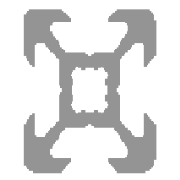
# Autodesk Inventor part: 2020 V-slot 100mm
Saved by Autodesk Inventor 2023 (Build 270158000, 158)
## iProperties
Created: 2023-08-13
Part Number: 2020 V-slot 100mm
Material: Generic
Description: STEP AP214
Document SubType Name: Modeling
Designer: Felix
Language: en-US
Size Designation: (Unnamed 1)
Categories: <MemberInstance><Categories><Category DisplayName="Structural Shapes" InternalName="089c4875-fa83-4c05-b084-43b9cc11f5ed" Mnemonic="GRDR"><CategoryParameter DisplayName="Mass per Length Unit" InternalName="0bb95a10-148f-4027-a459-38d7b056702a" Mnemonic="shpmass"/><CategoryParameter DisplayName="Section Area" InternalName="1ff91680-64b0-4202-b9a3-7fd3f94bba3b" Mnemonic="secarea"/><CategoryParameter DisplayName="Radius of Gyration (x)" InternalName="25778675-03e9-40c1-b6a8-4a9ed693320d" Mnemonic="gyrradx"/><CategoryParameter DisplayName="Torsional Rigidity Modulus" InternalName="26c1ec35-5026-4c63-ad0a-751cf684a536" Mnemonic="torrigmod"/><CategoryParameter DisplayName="Distance of the Center of Gravity X-X" InternalName="26c9bdb8-9c79-4b4f-a92e-8e197583c9c4" Mnemonic="grcendistX"/><CategoryParameter DisplayName="Legacy Member ID" InternalName="340afe4f-75d7-48d3-ab7d-943f3c3da468" Mnemonic="LegacyMemberID"/><CategoryParameter DisplayName="Base Length" InternalName="42e34263-8f20-4d0e-ad48-bf1385b87c24" Mnemonic="shplen"/><CategoryParameter DisplayName="Moment of Inertia (y)" InternalName="4b9f58ea-bced-460e-81ea-3d29ca5a49e3" Mnemonic="inermomy"/><CategoryParameter DisplayName="Moment of Inertia (x)" InternalName="4cd780bc-73d7-43ac-917a-579e5cbd684d" Mnemonic="inermomx"/><CategoryParameter DisplayName="Custom Base Point" InternalName="4f1d1b73-316d-484b-a3df-9cbabb16eb77" Mnemonic="shpBasePoint"/><CategoryParameter DisplayName="Shape Height" InternalName="50274e7d-5ac0-4796-92cb-c59e54983c67" Mnemonic="shpheig"/><CategoryParameter DisplayName="Section Module (y)" InternalName="59eaa5e9-d227-48dc-b6c1-6920f96e0f95" Mnemonic="secmody"/><CategoryParameter DisplayName="Section Designation" InternalName="5a64d034-428d-49c8-ba32-7619764de20f" Mnemonic="shpdes"/><CategoryParameter DisplayName="Section Module (x)" InternalName="72cfad18-cf51-4ed4-aaa7-c6b224f8419f" Mnemonic="secmodx"/><CategoryParameter DisplayName="Torsional Section Modulus" InternalName="7c55a8dc-8844-49f9-a867-cc677b30ec9a" Mnemonic="torsecmod"/><CategoryParameter DisplayName="Shape Width" InternalName="7c717d54-a18f-4666-b4d4-573cce22c62c" Mnemonic="shpwdth"/><CategoryParameter DisplayName="Second Shape Thickness" InternalName="9251a8e1-85fd-4e47-af99-afdb762317d9" Mnemonic="shpthick2"/><CategoryParameter DisplayName="FG Authored" InternalName="9c666724-f362-4ea7-ac62-f6a007de5c69" Mnemonic="shpFGAuto"/><CategoryParameter DisplayName="Distance of the Center of Gravity Y-Y" InternalName="bcc4fb17-7af4-436a-8f8c-d0aa3b0248c5" Mnemonic="grcendistY"/><CategoryParameter DisplayName="Radius of Gyration (y)" InternalName="bfa18ebe-1636-4dbe-8d42-b263e0b73184" Mnemonic="gyrrady"/><CategoryParameter DisplayName="Shape Thickness" InternalName="d109cf76-8eb4-42fc-9800-4409734adc67" Mnemonic="shpthick"/><CategoryParameter DisplayName="Coefficient of Shear Displacement" InternalName="de4c90c6-aaa8-468f-a335-6737b311b5d3" Mnemonic="shdispc"/><Category DisplayName="Other" InternalName="f02205ff-2390-476f-921c-0b3185f88e84" Mnemonic="OTHSHP"><CategoryParameter DisplayName="Moment of Inertia (y)" InternalName="044c654e-f649-48ac-84cc-650a29ae31ca" Mnemonic="inermomy"/><CategoryParameter DisplayName="Shape Thickness" InternalName="12b1a788-9233-48fd-a933-2df8ff42b15f" Mnemonic="shpthick"/><CategoryParameter DisplayName="Mass per Length Unit" InternalName="2fd289d6-9394-4d2d-97e6-6659d7d4551d" Mnemonic="shpmass"/><CategoryParameter DisplayName="Radius of Gyration (y)" InternalName="743e1dfe-1bba-408b-b985-cf752b207386" Mnemonic="gyrrady"/><CategoryParameter DisplayName="Section Module (y)" InternalName="88b8bff9-a616-4028-93d5-ed4f79680d13" Mnemonic="secmody"/><CategoryParameter DisplayName="Section Area" InternalName="c46ecdf8-b6eb-4db9-8b25-30258930c1e3" Mnemonic="secarea"/><CategoryParameter DisplayName="Section Module (x)" InternalName="cac70804-9d39-43bb-be17-56ea1f39a6c2" Mnemonic="secmodx"/><CategoryParameter DisplayName="Moment of Inertia (x)" InternalName="ec6737bc-264f-43ed-b0bd-f6d410c2718d" Mnemonic="inermomx"/><CategoryParameter DisplayName="Radius of Gyration (x)" InternalName="ee72c61e-565e-4fd6-b448-66e1e1abcb7e" Mnemonic="gyrradx"/></Category></Category><Category DisplayName="DataType" InternalName="23b78d0f-2648-40c6-8793-ca6db495c9e8" Mnemonic="DATATYPE"><CategoryParameter DisplayName="DisplayName" InternalName="05415f3d-3907-474b-a020-eb9d644f4cf3" Mnemonic="DISPLAYNAME"/><CategoryParameter DisplayName="Standard" InternalName="0c0a119c-1e12-4c84-803f-101930972f5e" Mnemonic="STANDARD"/><CategoryParameter DisplayName="Description" InternalName="13903e3d-64b1-4950-80da-f627842ea37f" Mnemonic="DESCRIPTION"/><CategoryParameter DisplayName="Designation" InternalName="2675968c-4ce5-49e0-a4f5-552d29089031" Mnemonic="DESIGNATION"/><CategoryParameter DisplayName="Default Row" InternalName="2af9ec52-faaa-4026-b378-f9fa4afca842" Mnemonic="DEFAULTROW"/><CategoryParameter DisplayName="Folder Name" InternalName="3f06958e-8713-4116-9be7-ed6184ecc97b" Mnemonic="FOLDERNAME"/><CategoryParameter DisplayName="Revision Guid" InternalName="45a75005-10b1-4dfc-8d6d-dfe629f0b93c" Mnemonic="REVISIONGUID"/><CategoryParameter DisplayName="FileName" InternalName="8b46a4cc-9585-4fed-90c3-899f57e09a73" Mnemonic="FILENAME"/><CategoryParameter DisplayName="StdsOrg" InternalName="8f5914e1-4693-403f-8ab5-d37768198c9d" Mnemonic="STDSORG"/><CategoryParameter DisplayName="Family Version" InternalName="914462f6-6e19-4b14-ba84-155b9680b1d0" Mnemonic="FAMILYREVISION"/><CategoryParameter DisplayName="Standard Revision" InternalName="91d5a463-65c2-4fde-b823-3b7fea5e8e17" Mnemonic="STANDARDREVISION"/><CategoryParameter DisplayName="Member Revision" InternalName="a65d44b9-392f-4f4f-857b-e4b3d54996fe" Mnemonic="MEMBERREVISION"/><CategoryParameter DisplayName="ClipFormat" InternalName="bc51e27b-3422-4e78-93ef-cec197ddf230" Mnemonic="CLIPFORMAT"/><CategoryParameter DisplayName="Manufacturer" InternalName="cd6c7a72-a28a-4e50-99a9-2c7f4e13e5ad" Mnemonic="MANUFACTURER"/><CategoryParameter DisplayName="InternalName" InternalName="cf1d0246-76d9-4b4a-8305-fa0409afb5c1" Mnemonic="INTERNALNAME"/><CategoryParameter DisplayName="IsMetric" InternalName="e2385c5b-1ea4-4823-96a8-8de651266ec3" Mnemonic="ISMETRIC"/><Category DisplayName="Part" InternalName="c0e0b642-3bcb-4cc8-9e80-f96d35c4afa4" Mnemonic="PART"><CategoryParameter DisplayName="Part Number" InternalName="016b6077-bfbe-49bd-92c9-d8d59c39c941" Mnemonic="PARTNUMBER"/><CategoryParameter DisplayName="Stock Number" InternalName="4dba7c1c-e26c-444e-836c-b08b433409a8" Mnemonic="STOCKNUMBER"/><CategoryParameter DisplayName="Material Key" InternalName="5c9a8adb-dd2b-4535-b97f-0a94a95fe41f" Mnemonic="MATERIALKEY"/><CategoryParameter DisplayName="Material" InternalName="818a152a-d3c3-49ca-80ee-df7d91421b8e" Mnemonic="MATERIAL"/></Category></Category></Categories><FamilyTemplate Id="3663_20220714183005_2020 V-slot 100mm"><FamilyTemplateParameters><FamilyTemplateParameter ObjectType="kUserParameterObject" ValueType="xs:double" Id="12" ObjectReferenceKey="LENGTH"/><FamilyTemplateParameter ObjectType="kPartComponentDefinitionObject" ValueType="xs:string" Id="23" SubObjectId="Material"/><FamilyTemplateParameter ObjectType="kPropertyObject" ValueType="xs:string" Id="26" ObjectReferenceKey="{32853F0F-3444-11d1-9E93-0060B03C1CA6}" SubObjectId="5"/><FamilyTemplateParameter ObjectType="kPropertyObject" ValueType="xs:string" Id="27" ObjectReferenceKey="{32853F0F-3444-11d1-9E93-0060B03C1CA6}" SubObjectId="52"/></FamilyTemplateParameters></FamilyTemplate><CategoryParameterMap><ParamToTemplateMap><ParamToTemplate CategoryParameter="//CategoryParameter[@InternalName='cf1d0246-76d9-4b4a-8305-fa0409afb5c1']" ConstantValue="2063e620-472c-4390-8693-845126e34f3a"/><ParamToTemplate CategoryParameter="//CategoryParameter[@InternalName='45a75005-10b1-4dfc-8d6d-dfe629f0b93c']" ConstantValue="7112f66b-08bf-44d2-881c-74bfb6beee39"/><ParamToTemplate CategoryParameter="//CategoryParameter[@InternalName='3f06958e-8713-4116-9be7-ed6184ecc97b']" ConstantValue="2020 V-slot"/><ParamToTemplate CategoryParameter="//CategoryParameter[@InternalName='8f5914e1-4693-403f-8ab5-d37768198c9d']" TemplateParameter="17"/><ParamToTemplate CategoryParameter="//CategoryParameter[@InternalName='0c0a119c-1e12-4c84-803f-101930972f5e']" TemplateParameter="18"/><ParamToTemplate CategoryParameter="//CategoryParameter[@InternalName='91d5a463-65c2-4fde-b823-3b7fea5e8e17']" TemplateParameter="19"/><ParamToTemplate CategoryParameter="//CategoryParameter[@InternalName='cd6c7a72-a28a-4e50-99a9-2c7f4e13e5ad']" TemplateParameter="20"/><ParamToTemplate CategoryParameter="//CategoryParameter[@InternalName='13903e3d-64b1-4950-80da-f627842ea37f']" ConstantValue="STEP AP214"/><ParamToTemplate CategoryParameter="//CategoryParameter[@InternalName='05415f3d-3907-474b-a020-eb9d644f4cf3']" ConstantValue="2020 V-slot"/><ParamToTemplate CategoryParameter="//CategoryParameter[@InternalName='914462f6-6e19-4b14-ba84-155b9680b1d0']" ConstantValue="11"/><ParamToTemplate CategoryParameter="//CategoryParameter[@InternalName='bc51e27b-3422-4e78-93ef-cec197ddf230']" ConstantValue="CF_INVENTOR.STDPARTS"/><ParamToTemplate CategoryParameter="//CategoryParameter[@InternalName='e2385c5b-1ea4-4823-96a8-8de651266ec3']" ConstantValue="true"/><ParamToTemplate CategoryParameter="//CategoryParameter[@InternalName='2af9ec52-faaa-4026-b378-f9fa4afca842']" ConstantValue="1"/><ParamToTemplate CategoryParameter="//CategoryParameter[@InternalName='9c666724-f362-4ea7-ac62-f6a007de5c69']" ConstantValue="1"/><ParamToTemplate CategoryParameter="//CategoryParameter[@InternalName='8b46a4cc-9585-4fed-90c3-899f57e09a73']" ConstantValue="1"/><ParamToTemplate CategoryParameter="//CategoryParameter[@InternalName='a65d44b9-392f-4f4f-857b-e4b3d54996fe']" ConstantValue="1e38da75-13bc-491b-9e5a-c7c1421ad0a4"/><ParamToTemplate CategoryParameter="//CategoryParameter[@InternalName='a65d44b9-392f-4f4f-857b-e4b3d54996fe']" ConstantValue="1e38da75-13bc-491b-9e5a-c7c1421ad0a4"/><ParamToTemplate CategoryParameter="//CategoryParameter[@InternalName='2675968c-4ce5-49e0-a4f5-552d29089031']" TemplateParameter="27"/><ParamToTemplate CategoryParameter="//CategoryParameter[@InternalName='42e34263-8f20-4d0e-ad48-bf1385b87c24']" TemplateParameter="12"/><ParamToTemplate CategoryParameter="//CategoryParameter[@InternalName='818a152a-d3c3-49ca-80ee-df7d91421b8e']" TemplateParameter="23"/><ParamToTemplate CategoryParameter="//CategoryParameter[@InternalName='016b6077-bfbe-49bd-92c9-d8d59c39c941']" TemplateParameter="26"/></ParamToTemplateMap></CategoryParameterMap></MemberInstance>
Density: 1 g/cm^3
Appearance: Default
IsCustomPart: 1
_CCFamilyDisplayName: 2020 V-slot - STEP AP214
_FrameMemberDoc: Frame Member File
_Version: 25.0.0
_GetPNFromCC: 1
Title: 2020 V-slot 100mm.STEP
Author: Felix
Sending System: SolidWorks 2018
Preprocessor: SwSTEP 2.0
G_L: 520,000 mm
G_W: 20,000 mm
G_H: 20,000 mm
+3BCE196E-394D-4133-8DB2-D45BFDC7B2EE+CUTDETAIL1: Corner Joint
+C0951EA9-A871-42D9-A546-154018CCC8EC+CUTDETAIL2: Corner Joint
Autodesk Inventor part; units mm, degrees
ref_plane "YZ Plane" through (0, 0, 0) normal (1, 0, 0) x (0, 1, 0)
ref_plane "XZ Plane" through (0, 0, 0) normal (0, 1, 0) x (-1, 0, 0)
ref_plane "XY Plane" through (0, 0, 0) normal (0, 0, 1) x (1, 0, 0)
ref_plane "Work Plane5" through (12.8, 0, 50) normal (0, 0, 1) x (1, 0, 0)
sketch "Sketch" plane through (12.8, 0, 50) normal (0, 0, 1) x (1, 0, 0)
  arc A0 (1.7, 2.7322) -> (1.5536, 3.0858) centre (1.2, 2.7322) ccw
  line L0 (1.7, 2.7322) -> (1.7, 2)
  arc A1 (1.2, 1.5) -> (1.7, 2) centre (1.2, 2) ccw
  line L1 (1.2, 1.5) -> (-1.2, 1.5)
  line L2 (-1.2, 1.5) -> (-1.2, 1.2)
  line L3 (-1.2, 1.2) -> (0, 0)
  line L4 (0, 0) -> (4.2, 0)
  arc A2 (4.2, 0) -> (5.7, 1.5) centre (4.2, 1.5) ccw
  line L5 (5.7, 1.5) -> (5.7, 5.7)
  line L6 (5.7, 5.7) -> (4.5, 6.9)
  line L7 (4.5, 6.9) -> (4.2, 6.9)
  line L8 (4.2, 6.9) -> (4.2, 4.5)
  arc A3 (3.7, 4) -> (4.2, 4.5) centre (3.7, 4.5) ccw
  line L9 (3.7, 4) -> (2.9678, 4)
  arc A4 (2.6142, 4.1464) -> (2.9678, 4) centre (2.9678, 4.5) ccw
  line L10 (2.6142, 4.1464) -> (0.3464, 6.4142)
  arc A5 (0.2, 6.7678) -> (0.3464, 6.4142) centre (0.7, 6.7678) ccw
  line L11 (0.2, 6.7678) -> (0.2, 9.0464)
  arc A6 (0.2, 9.0464) -> (0.1732, 9.1464) centre (0, 9.0464) ccw
  line L12 (0.1732, 9.1464) -> (-0.2619, 9.9)
  arc A7 (-0.2619, 10.1) -> (-0.2619, 9.9) centre (-0.0887, 10) ccw
  line L13 (-0.2619, 10.1) -> (0.1732, 10.8536)
  arc A8 (0.1732, 10.8536) -> (0.2, 10.9536) centre (0, 10.9536) ccw
  line L14 (0.2, 10.9536) -> (0.2, 13.2322)
  arc A9 (0.3464, 13.5858) -> (0.2, 13.2322) centre (0.7, 13.2322) ccw
  line L15 (0.3464, 13.5858) -> (2.6142, 15.8536)
  arc A10 (2.9678, 16) -> (2.6142, 15.8536) centre (2.9678, 15.5) ccw
  line L16 (2.9678, 16) -> (3.7, 16)
  arc A11 (4.2, 15.5) -> (3.7, 16) centre (3.7, 15.5) ccw
  line L17 (4.2, 15.5) -> (4.2, 13.1)
  line L18 (4.2, 13.1) -> (4.5, 13.1)
  line L19 (4.5, 13.1) -> (5.7, 14.3)
  line L20 (5.7, 14.3) -> (5.7, 18.5)
  arc A12 (5.7, 18.5) -> (4.2, 20) centre (4.2, 18.5) ccw
  line L21 (4.2, 20) -> (0, 20)
  line L22 (0, 20) -> (-1.2, 18.8)
  line L23 (-1.2, 18.8) -> (-1.2, 18.5)
  line L24 (-1.2, 18.5) -> (1.2, 18.5)
  arc A13 (1.7, 18) -> (1.2, 18.5) centre (1.2, 18) ccw
  line L25 (1.7, 18) -> (1.7, 17.2678)
  arc A14 (1.5536, 16.9142) -> (1.7, 17.2678) centre (1.2, 17.2678) ccw
  line L26 (1.5536, 16.9142) -> (-0.7142, 14.6464)
  arc A15 (-1.0678, 14.5) -> (-0.7142, 14.6464) centre (-1.0678, 15) ccw
  line L27 (-1.0678, 14.5) -> (-3.3464, 14.5)
  arc A16 (-3.3464, 14.5) -> (-3.4464, 14.4732) centre (-3.3464, 14.3) ccw
  line L28 (-3.4464, 14.4732) -> (-4.2, 14.0381)
  arc A17 (-4.4, 14.0381) -> (-4.2, 14.0381) centre (-4.3, 14.2113) ccw
  line L29 (-4.4, 14.0381) -> (-5.1536, 14.4732)
  arc A18 (-5.1536, 14.4732) -> (-5.2536, 14.5) centre (-5.2536, 14.3) ccw
  line L30 (-5.2536, 14.5) -> (-7.5322, 14.5)
  arc A19 (-7.8858, 14.6464) -> (-7.5322, 14.5) centre (-7.5322, 15) ccw
  line L31 (-7.8858, 14.6464) -> (-10.1536, 16.9142)
  arc A20 (-10.3, 17.2678) -> (-10.1536, 16.9142) centre (-9.8, 17.2678) ccw
  line L32 (-10.3, 17.2678) -> (-10.3, 18)
  arc A21 (-9.8, 18.5) -> (-10.3, 18) centre (-9.8, 18) ccw
  line L33 (-9.8, 18.5) -> (-7.4, 18.5)
  line L34 (-7.4, 18.5) -> (-7.4, 18.8)
  line L35 (-7.4, 18.8) -> (-8.6, 20)
  line L36 (-8.6, 20) -> (-12.8, 20)
  arc A22 (-12.8, 20) -> (-14.3, 18.5) centre (-12.8, 18.5) ccw
  line L37 (-14.3, 18.5) -> (-14.3, 14.3)
  line L38 (-14.3, 14.3) -> (-13.1, 13.1)
  line L39 (-13.1, 13.1) -> (-12.8, 13.1)
  line L40 (-12.8, 13.1) -> (-12.8, 15.5)
  arc A23 (-12.3, 16) -> (-12.8, 15.5) centre (-12.3, 15.5) ccw
  line L41 (-12.3, 16) -> (-11.5678, 16)
  arc A24 (-11.2142, 15.8536) -> (-11.5678, 16) centre (-11.5678, 15.5) ccw
  line L42 (-11.2142, 15.8536) -> (-8.9464, 13.5858)
  arc A25 (-8.8, 13.2322) -> (-8.9464, 13.5858) centre (-9.3, 13.2322) ccw
  line L43 (-8.8, 13.2322) -> (-8.8, 10.9536)
  arc A26 (-8.8, 10.9536) -> (-8.7732, 10.8536) centre (-8.6, 10.9536) ccw
  line L44 (-8.7732, 10.8536) -> (-8.3381, 10.1)
  arc A27 (-8.3381, 9.9) -> (-8.3381, 10.1) centre (-8.5113, 10) ccw
  line L45 (-8.3381, 9.9) -> (-8.7732, 9.1464)
  arc A28 (-8.7732, 9.1464) -> (-8.8, 9.0464) centre (-8.6, 9.0464) ccw
  line L46 (-8.8, 9.0464) -> (-8.8, 6.7678)
  arc A29 (-8.9464, 6.4142) -> (-8.8, 6.7678) centre (-9.3, 6.7678) ccw
  line L47 (-8.9464, 6.4142) -> (-11.2142, 4.1464)
  arc A30 (-11.5678, 4) -> (-11.2142, 4.1464) centre (-11.5678, 4.5) ccw
  line L48 (-11.5678, 4) -> (-12.3, 4)
  arc A31 (-12.8, 4.5) -> (-12.3, 4) centre (-12.3, 4.5) ccw
  line L49 (-12.8, 4.5) -> (-12.8, 6.9)
  line L50 (-12.8, 6.9) -> (-13.1, 6.9)
  line L51 (-13.1, 6.9) -> (-14.3, 5.7)
  line L52 (-14.3, 5.7) -> (-14.3, 1.5)
  arc A32 (-14.3, 1.5) -> (-12.8, 0) centre (-12.8, 1.5) ccw
  line L53 (-12.8, 0) -> (-8.6, 0)
  line L54 (-8.6, 0) -> (-7.4, 1.2)
  line L55 (-7.4, 1.2) -> (-7.4, 1.5)
  line L56 (-7.4, 1.5) -> (-9.8, 1.5)
  arc A33 (-10.3, 2) -> (-9.8, 1.5) centre (-9.8, 2) ccw
  line L57 (-10.3, 2) -> (-10.3, 2.7322)
  arc A34 (-10.1536, 3.0858) -> (-10.3, 2.7322) centre (-9.8, 2.7322) ccw
  line L58 (-10.1536, 3.0858) -> (-7.8858, 5.3536)
  arc A35 (-7.5322, 5.5) -> (-7.8858, 5.3536) centre (-7.5322, 5) ccw
  line L59 (-7.5322, 5.5) -> (-5.2536, 5.5)
  arc A36 (-5.2536, 5.5) -> (-5.1536, 5.5268) centre (-5.2536, 5.7) ccw
  line L60 (-5.1536, 5.5268) -> (-4.4, 5.9619)
  arc A37 (-4.2, 5.9619) -> (-4.4, 5.9619) centre (-4.3, 5.7887) ccw
  line L61 (-4.2, 5.9619) -> (-3.4464, 5.5268)
  arc A38 (-3.4464, 5.5268) -> (-3.3464, 5.5) centre (-3.3464, 5.7) ccw
  line L62 (-3.3464, 5.5) -> (-1.0678, 5.5)
  arc A39 (-0.7142, 5.3536) -> (-1.0678, 5.5) centre (-1.0678, 5) ccw
  line L63 (-0.7142, 5.3536) -> (1.5536, 3.0858)
  line L64 (-6.7453, 8.7418) -> (-7.2922, 8.0901)
  arc A40 (-6.7453, 11.2582) -> (-6.7453, 8.7418) centre (-4.3, 10) ccw
  line L65 (-7.2922, 11.9099) -> (-6.7453, 11.2582)
  arc A41 (-6.2139, 12.9896) -> (-7.2922, 11.9099) centre (-4.3, 10) ccw
  line L66 (-5.5582, 12.4453) -> (-6.2139, 12.9896)
  arc A42 (-3.0418, 12.4453) -> (-5.5582, 12.4453) centre (-4.3, 10) ccw
  line L67 (-2.3861, 12.9896) -> (-3.0418, 12.4453)
  arc A43 (-1.3078, 11.9099) -> (-2.3861, 12.9896) centre (-4.3, 10) ccw
  line L68 (-1.8547, 11.2582) -> (-1.3078, 11.9099)
  arc A44 (-1.8547, 8.7418) -> (-1.8547, 11.2582) centre (-4.3, 10) ccw
  line L69 (-1.3078, 8.0901) -> (-1.8547, 8.7418)
  arc A45 (-2.3861, 7.0104) -> (-1.3078, 8.0901) centre (-4.3, 10) ccw
  line L70 (-3.0418, 7.5547) -> (-2.3861, 7.0104)
  arc A46 (-5.5582, 7.5547) -> (-3.0418, 7.5547) centre (-4.3, 10) ccw
  line L71 (-6.2139, 7.0104) -> (-5.5582, 7.5547)
  arc A47 (-7.2922, 8.0901) -> (-6.2139, 7.0104) centre (-4.3, 10) ccw
  constraints: 144 end point, 96 point on circle, 48 centre point, 20 horizontal, 16 vertical, 253 other
ref_plane "Start Plane" through (12.8, 0, 50) normal (0, 0, 1) x (1, 0, 0)
ref_plane "End Plane" through (12.8, 0, 570) normal (0, 0, 1) x (1, 0, 0)
extrude "Body" add sketch "Sketch" along normal up to surface (520 mm away) from surface at 0
sketch "Sketch8" plane through (12.8, 0, 50) normal (0, 0, 1) x (1, 0, 0)
  line L0 (0, 0) -> (10, 0)
ref_plane "Work Plane10" through (12.8, 0, 50) normal (0, -1, 0) x (1, 0, 0)
sketch "Sketch9" plane through (12.8, 0, 50) normal (0, -1, 0) x (1, 0, 0)
  line L0 (-2, 0) -> (12, 0)
  line L1 (-2, 520) -> (12, 520)
  dimension "d16" = 520
  measures "d16" distance between parallel lines of L0 L1
ref_plane "Work Plane11" through (8.5, 0, 570) normal (0, 0, 1) x (1, 0, 0)
split "Split1" plane through (8.5, 0, 570) removes the side toward (0, 0, 1)
ref_plane "Work Plane12" through (8.5, -714, 50) normal (0, 0, -1) x (-1, 0, 0)
split "Split2" plane through (8.5, -714, 50) removes the side toward (0, 0, -1)
equation "\"G_OFFSET_START\" = 0"
equation "\"G_OFFSET_END\" = 0"
equation "\"G_L\" = d16"
equation "\"G_OFFSET_START1\" = 0"
equation "\"G_OFFSET_END1\" = 0"
body "Solid2"
